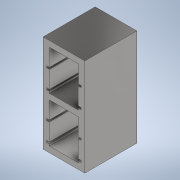
# Autodesk Inventor part: Rack
Saved by Autodesk Inventor 2021 (Build 250183000, 183)
## iProperties
Created: 2023-04-05
Part Number: Rack
Material: Generic
Document SubType Name: Modeling
Designer: EF0481
Density: 1 g/cm^3
Appearance: Steel - Polished
Author: EF0481
Autodesk Inventor part; units mm, degrees
ref_plane "YZ Plane" through (0, 0, 0) normal (1, 0, 0) x (0, 1, 0)
ref_plane "XZ Plane" through (0, 0, 0) normal (0, 1, 0) x (-1, 0, 0)
ref_plane "XY Plane" through (0, 0, 0) normal (0, 0, 1) x (1, 0, 0)
sketch "Sketch7" plane through (0, 0, 0) normal (0, 0, 1) x (1, 0, 0)
  line L0 (0, 0) -> (72, 0)
  line L1 (0, 82.9989) -> (0, 0)
  line L2 (10.6826, 79) -> (60.6826, 79)
  line L3 (10.6826, 79) -> (10.6826, 49)
  line L4 (10.6826, 49) -> (5.6826, 49)
  line L5 (5.6826, 49) -> (5.6826, 46)
  line L6 (5.6826, 46) -> (10.6826, 46)
  line L7 (10.6826, 46) -> (10.6826, 16)
  line L8 (10.6826, 16) -> (5.6826, 16)
  line L9 (5.6826, 16) -> (5.6826, 13)
  line L10 (5.6826, 13) -> (10.6826, 13)
  line L11 (10.6826, 13) -> (10.6826, 10)
  line L12 (10.6826, 10) -> (60.6826, 10)
  line L13 (60.6826, 49) -> (65.6826, 49)
  line L14 (65.6826, 49) -> (65.6826, 46)
  line L15 (65.6826, 46) -> (60.6826, 46)
  line L16 (60.6826, 16) -> (65.6826, 16)
  line L17 (65.6826, 16) -> (65.6826, 13)
  line L18 (65.6826, 13) -> (60.6826, 13)
  line L19 (60.6826, 79) -> (60.6826, 49)
  line L20 (60.6826, 46) -> (60.6826, 25.2456)
  line L21 (60.6826, 10) -> (60.6826, 13)
  line L22 (60.6826, 16) -> (60.6826, 25.2456)
  line L23 (72, 82.9992) -> (72, 0)
  line L24 (0, 82.9989) -> (0, 167.9989)
  line L25 (0, 167.9989) -> (72, 167.9989)
  line L26 (72, 167.9989) -> (72, 82.9992)
  line L27 (10.6362, 89) -> (60.6362, 89)
  line L28 (11.0233, 157.9989) -> (61.0233, 157.9989)
  line L29 (11.0233, 157.9989) -> (11.0233, 127.9989)
  line L30 (11.0233, 127.9989) -> (6.0233, 127.9989)
  line L31 (6.0233, 127.9989) -> (6.0233, 124.9989)
  line L32 (6.0233, 124.9989) -> (11.0233, 124.9989)
  line L33 (11.0233, 124.9989) -> (11.0233, 94.9989)
  line L34 (11.0233, 94.9989) -> (6.0233, 95)
  line L35 (6.0233, 95) -> (6.0233, 92)
  line L36 (6.0233, 92) -> (10.6362, 92)
  line L37 (10.6362, 92) -> (10.6362, 89)
  line L38 (61.0233, 127.9992) -> (65.683, 127.9992)
  line L39 (65.683, 127.9992) -> (65.683, 125)
  line L40 (65.683, 125) -> (60.683, 125)
  line L41 (60.683, 95) -> (65.683, 95)
  line L42 (65.683, 95) -> (65.683, 92)
  line L43 (65.683, 92) -> (60.6362, 92)
  line L44 (11.0233, 157.9989) -> (11.0233, 127.9989)
  line L45 (11.0233, 124.9989) -> (11.0233, 94.9989)
  line L46 (10.6362, 92) -> (10.6362, 89)
  line L47 (60.6362, 92) -> (60.6362, 89)
  line L48 (61.0233, 157.9989) -> (61.0233, 127.9992)
  line L49 (60.683, 125) -> (60.683, 95)
  dimension "d86" = 30
  dimension "d87" = 5
  dimension "d88" = 3
  dimension "d90" = 30
  dimension "d91" = 5
  dimension "d92" = 3
  dimension "d93" = 3
  dimension "d94" = 50
  dimension "d95" = 50
  dimension "d98" = 85
  dimension "d99" = 72
  dimension "d100" = 69
  dimension "d101" = 50
  dimension "d103" = 30
  dimension "d104" = 5
  dimension "d105" = 3
  dimension "d106" = 30
  dimension "d107" = 5
  dimension "d108" = 3
  dimension "d109" = 4.6129
  dimension "d110" = 10
  dimension "d111" = 10
  dimension "d112" = 10
  dimension "d113" = 3
  constraints: 100 end point, 23 perpendicular, 6 horizontal, 5 vertical, 4 point on line
  measures "d86" distance of L2.start L3.end
  measures "d87" distance of L3.end L4.end
  measures "d88" distance of L4.end L5.end
  measures "d90" distance of L6.end L7.end
  measures "d91" distance of L7.end L8.end
  measures "d92" distance of L8.end L9.end
  measures "d93" distance of L10.end L11.end
  measures "d94" distance of L2.start L2.end
  measures "d95" distance of L11.end L12.end
  measures "d98" distance of L1.start L24.end
  measures "d99" distance of L24.end L25.end
  measures "d100" distance of L28.start L27.start
  measures "d101" distance of L27.start L27.end
  measures "d103" distance of L28.start L29.end
  measures "d104" distance of L29.end L30.end
  measures "d105" distance of L30.end L31.end
  measures "d106" distance of L32.end L33.end
  measures "d107" distance of L33.end L34.end
  measures "d108" distance of L34.end L35.end
  measures "d109" distance of L35.end L36.end
  measures "d110" distance between parallel lines of L2 L27
  measures "d111" distance between parallel lines of L0 L12
  measures "d112" distance between parallel lines of L28 L25
  measures "d113" distance between parallel lines of L27 L36
extrude "Extrusion5" add sketch "Sketch7" against normal blind 90
body "Solid2"
